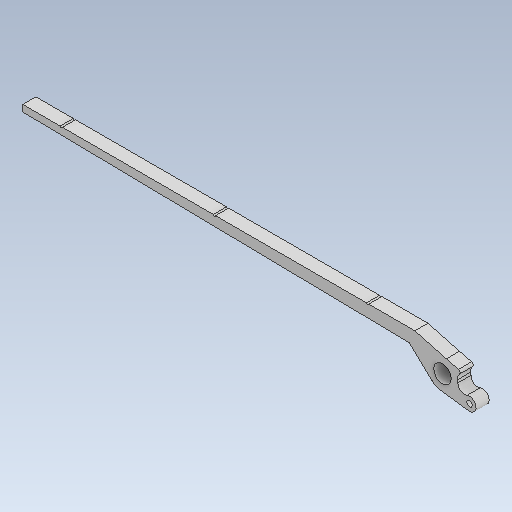
# Autodesk Inventor part: シールド先端棒
Saved by Autodesk Inventor 2020 (Build 240168000, 168)
## iProperties
Created: 2020-02-13
Part Number: シールド先端棒
Material: 一般
Document SubType Name: Modeling
Designer: tanjihayato
Density: 1 g/cm^3
Appearance: 既定
Mass: 6.33546 g
Surface Area: 49.2691 cm^2
Volume: 6.33546 cm^3
Author: tanjihayato
Autodesk Inventor part; units mm, degrees
ref_plane "YZ Plane" through (0, 0, 0) normal (1, 0, 0) x (0, 1, 0)
ref_plane "XZ Plane" through (0, 0, 0) normal (0, 1, 0) x (-1, 0, 0)
ref_plane "XY Plane" through (0, 0, 0) normal (0, 0, 1) x (1, 0, 0)
sketch "スケッチ1" plane through (0, 0, 0) normal (0, 0, 1) x (1, 0, 0)
  line L0 (0, 0) -> (0, -3)
  line L1 (0, 0) -> (-15, 0)
  line L2 (-15, 0) -> (-15, -3)
  line L3 (-15, -3) -> (-30, -3)
  line L4 (-30, -3) -> (-30, 0)
  line L5 (-30, 0) -> (-45, 0)
  line L6 (-45, 0) -> (-45, -3)
  line L7 (-245.5996, 0) -> (-66.4062, 0)
  line L8 (-66.4062, 0) -> (-51.9242, -3.906)
  line L9 (-245.5996, 0) -> (-245.5996, -3)
  line L10 (-245.5996, -3) -> (-68.9626, -6)
  line L11 (-68.9626, -6) -> (-58.5737, -15.799)
  circle A0 centre (-53.7535, -10.6886) radius 4.025
  circle A1 centre (-53.7535, -10.6886) radius 1.5
  line L12 (0, -3) -> (0, -9)
  arc A2 (-54.2694, -3.6826) -> (-51.0532, -17.1739) centre (-53.7535, -10.6886) ccw
  line L13 (-54.2694, -3.6826) -> (-45, -3)
  line L14 (-51.0532, -17.1739) -> (-31.4218, -9)
  line L15 (-31.4218, -9) -> (0, -9)
  arc A3 (-46.7293, -10.7926) -> (-42.5418, -13.63) centre (-43.7046, -10.8374) ccw
  circle A4 centre (-43.7046, -10.8374) radius 1.5
  line L16 (-54.6828, -17.6519) -> (-41.7856, -19.3732)
  arc A5 (-41.7856, -19.3732) -> (-42.5418, -13.63) centre (-41.3887, -16.3996) ccw
  arc A6 (-58.5737, -15.799) -> (-54.6828, -17.6519) centre (-53.7535, -10.6886) ccw
  arc A7 (-46.7293, -10.7926) -> (-51.9242, -3.906) centre (-53.7535, -10.6886) ccw
  line L17 (-42, -3) -> (-33, -3)
  line L18 (-33, -3) -> (-33, -6)
  line L19 (-33, -6) -> (-42, -6)
  line L20 (-42, -6) -> (-42, -3)
  line L21 (-12, -3) -> (-3, -3)
  line L22 (-3, -3) -> (-3, -6)
  line L23 (-3, -6) -> (-12, -6)
  line L24 (-12, -6) -> (-12, -3)
  circle A8 centre (-40.95, -3) radius 1.05
  circle A9 centre (-34.05, -3) radius 1.05
  circle A10 centre (-34.05, -6) radius 1.05
  circle A11 centre (-40.95, -6) radius 1.05
  circle A12 centre (-10.95, -3) radius 1.05
  circle A13 centre (-4.05, -3) radius 1.05
  circle A14 centre (-4.05, -6) radius 1.05
  circle A15 centre (-10.95, -6) radius 1.05
  circle A16 centre (-28.95, -3) radius 1.05
  circle A17 centre (-16.05, -3) radius 1.05
  circle A18 centre (-41.3887, -16.3996) radius 1.25
  line L25 (-15.5802, -9) -> (-15.5802, -14)
  line L26 (-15.5802, -14) -> (-4.3492, -14)
  line L27 (-4.3492, -14) -> (-4.3492, -12)
  line L28 (-4.3492, -12) -> (-11.5802, -12)
  arc A19 (-11.5802, -9) -> (-11.5802, -12) centre (-11.5802, -10.5) ccw
  line L29 (-43.7046, -10.8374) -> (-53.7535, -10.6886)
  line L30 (-53.7535, -10.6886) -> (-43.8314, -9.0902)
  arc A20 (-43.0841, -6.159) -> (-46.8179, -9.5713) centre (-43.8314, -9.0902) ccw
  line L31 (-52.0181, -3.8813) -> (-43.0841, -6.159)
  circle A21 centre (-88, 0) radius 0.5
  circle A22 centre (-158, 0) radius 0.5
  circle A23 centre (-228, 0) radius 0.5
  point P0 (-5.1, -6)
  point P1 (-9.9, -6)
  point P2 (-12, -6)
  point P3 (-9.9, -3)
  point P4 (-5.1, -3)
  point P5 (-33, -3)
  point P6 (-33, -6)
  point P7 (-35.1, -6)
  point P8 (-39.9, -6)
  point P9 (-42, -6)
  point P10 (-42, -3)
  point P11 (-39.9, -3)
  point P12 (-35.1, -3)
  point P13 (-17.1, -3)
  point P14 (-27.9, -3)
  point P15 (-58.5737, -15.799)
  point P16 (-54.6828, -17.6519)
  point P17 (-51.9709, -3.8934)
  point P18 (-46.8179, -9.5713)
  point P19 (-87.5, 0)
  point P20 (-88.5, 0)
  point P21 (-157.5, 0)
  point P22 (-158.5, 0)
  point P23 (-227.5, 0)
  point P24 (-228.5, 0)
  dimension "d0" = 3
  dimension "d1" = 15
  dimension "d2" = 3
  dimension "d3" = 15
  dimension "d4" = 15
  dimension "d5" = 3
  dimension "d6" = 3
  dimension "d7" = 8.05
  dimension "d8" = 3
  dimension "d9" = 6
  dimension "d10" = 6
  dimension "d11" = 6.05
  dimension "d12" = 3
  dimension "d13" = 9
  dimension "d14" = 3
  dimension "d15" = 9
  dimension "d16" = 3
  dimension "d17" = 3
  dimension "d18" = 3
  dimension "d19" = 3
  dimension "d20" = 3
  dimension "d21" = 3
  dimension "d22" = 2.1
  dimension "d23" = 2.1
  dimension "d24" = 2.1
  dimension "d25" = 2.1
  dimension "d26" = 2.1
  dimension "d27" = 2.1
  dimension "d28" = 2.1
  dimension "d29" = 2.1
  dimension "d30" = 2.1
  dimension "d31" = 2.1
  dimension "d32" = 2.5
  dimension "d33" = 3
  dimension "d34" = 3
  dimension "d35" = 2
  dimension "d36" = 4
  dimension "d39" = 10
  dimension "d42" = 1
  dimension "d43" = 43
  dimension "d44" = 1
  dimension "d45" = 1
  dimension "d46" = 70
  dimension "d47" = 70
  constraints: 65 end point, 25 tangent, 24 centre point, 20 point on line, 15 point on circle, 7 perpendicular, 6 coincident, 6 vertical, 5 horizontal, 4 parallel, 2 collinear, 1 equal length, 3 other
  measures "d0" distance of L0.start L0.end
  measures "d1" distance of L0.start L1.end
  measures "d2" distance of L1.end L2.end
  measures "d3" distance of L2.end L3.end
  measures "d4" distance of L4.end L5.end
  measures "d5" distance of L5.end L6.end
  measures "d6" distance of L7.start L9.end
  measures "d7" diameter of A0
  measures "d8" diameter of A1
  measures "d9" distance of L0.end L12.end
  measures "d10" distance from line of L7 L10.end
  measures "d11" diameter of A3
  measures "d12" diameter of A4
  measures "d13" distance of L18.end L19.end
  measures "d14" distance of L17.end L18.end
  measures "d15" distance of L22.end L23.end
  measures "d16" distance of L21.end L22.end
  measures "d17" radial gap between concentric circles of A2 A0
  measures "d18" radial gap between concentric circles of A6 A0
  measures "d19" radial gap between concentric circles of A7 A0
  measures "d20" distance between parallel lines of L18 L4
  measures "d21" distance between parallel lines of L24 L2
  measures "d22" diameter of A8
  measures "d23" diameter of A9
  measures "d24" diameter of A10
  measures "d25" diameter of A11
  measures "d26" diameter of A12
  measures "d27" diameter of A13
  measures "d28" diameter of A14
  measures "d29" diameter of A15
  measures "d30" diameter of A16
  measures "d31" diameter of A17
  measures "d32" diameter of A18
  measures "d33" radius of A5
  measures "d34" distance between parallel lines of L28 L15
  measures "d35" distance between parallel lines of L26 L28
  measures "d36" distance from line of L25 A19.centre
  measures "d39" angle of L30 L29
  measures "d42" diameter of A21
  measures "d43" distance from line of A21.centre L6
  measures "d44" diameter of A22
  measures "d45" diameter of A23
  measures "d46" distance of A22.centre A21.centre
  measures "d47" distance of A23.centre A22.centre
extrude "押し出し1" add sketch "スケッチ1" along normal blind 6 contours A5 L16 A2 L14 | L14 A2 L13 L8 A7 L30 A0 L29 A3 | L29 A0 L30 A7 | A7 L31 A20 | L11 L10 L9 L7 A23 A22 A21 L8 L13 A2
fillet "フィレット1" radius 1 1 edges at (-43.0841, -6.159, 3)
